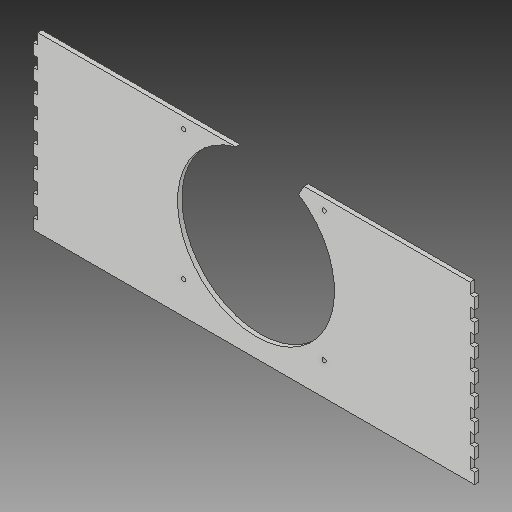
# Autodesk Inventor part: Stenka
Saved by Autodesk Inventor 2019 (Build 230136000, 136)
## iProperties
Created: 2022-06-29
Part Number: Stenka
Material: Типовые
Document SubType Name: Modeling
Designer: korsh
Density: 1 g/cm^3
Appearance: По умолчанию
Author: korsh
Autodesk Inventor part; units mm, degrees
ref_plane "YZ Plane" through (0, 0, 0) normal (1, 0, 0) x (0, 1, 0)
ref_plane "XZ Plane" through (0, 0, 0) normal (0, 1, 0) x (-1, 0, 0)
ref_plane "XY Plane" through (0, 0, 0) normal (0, 0, 1) x (1, 0, 0)
sketch "Эскиз1" plane through (0, 0, 0) normal (0, 0, 1) x (1, 0, 0)
  line L0 (-77, 69.9999) -> (-77, -70.0001) projected
  line L1 (-202, 69.9999) -> (198, 69.9999)
  line L2 (198, 69.9999) -> (198, -70.0001)
  line L3 (198, -70.0001) -> (-202, -70.0001)
  line L4 (-202, -70.0001) -> (-202, 69.9999)
  line L5 (73, -70.0001) -> (73, 69.9999) projected
  arc A0 (-18.8748, 69.9999) -> (-18.8744, -70.0001) centre (0, 0) ccw projected
  arc A1 (18.8744, -70.0001) -> (39.3067, 60.9199) centre (0, 0) ccw projected
  line L6 (44.4476, 69.9999) -> (36.592, 56.1251) projected
  line L7 (73, 69.9999) -> (44.4476, 69.9999) projected
  circle A2 centre (63, 59.9999) radius 2 projected
  circle A3 centre (-67, 59.9999) radius 2 projected
  circle A4 centre (-67, -60.0001) radius 2 projected
  circle A5 centre (63, -60.0001) radius 2 projected
  line L8 (44.4476, 69.9999) -> (73, 69.9999)
  point P0 (0, 0)
  dimension "d0" = 140
  dimension "d1" = 400
  dimension "d2" = 150
  dimension "d3" = 125
  constraints: 10 end point, 3 equal length, 1 horizontal, 1 perpendicular, 2 other
  measures "d0" distance of L3.end L1.start
  measures "d1" distance between parallel lines of L2 L4
  measures "d2" distance between parallel lines of L5 L0
  measures "d3" distance between parallel lines of L4 L0
extrude "Выдавливание1" add sketch "Эскиз1" along normal blind 4
sketch "Эскиз2" plane through (0, 0, 4) normal (0, 0, 1) x (1, 0, 0)
  line L0 (-202, -70.0001) -> (198, -70.0001) projected
  line L1 (198, -70.0001) -> (198, -90.0001)
  arc A0 (-18.8744, -70.0001) -> (18.8744, -70.0001) centre (0, 0) ccw projected
  line L2 (-202, -70.0001) -> (198, -70.0001) projected
  line L3 (-202, 69.9999) -> (-202, -70.0001) projected
  line L4 (-202, -70.0001) -> (-202, -90.0001)
  line L5 (-202, -90.0001) -> (198, -90.0001)
  point P0 (0, 0)
  dimension "d6" = 20
  constraints: 6 end point, 2 vertical, 1 perpendicular
  measures "d6" distance of L0.end L1.end
extrude "Выдавливание2" add sketch "Эскиз2" against normal blind 4
sketch "Эскиз3" plane through (0, 0, 4) normal (0, 0, 1) x (1, 0, 0)
  line L0 (198, 69.9999) -> (198, -90.0001) projected
  line L1 (-202, 69.9999) -> (-202, -90.0001) projected
  line L2 (198, -90.0001) -> (-202, -90.0001) projected
  line L3 (198, -90.0001) -> (202, -90.0001)
  line L4 (202, -90.0001) -> (202, -80.0001)
  line L5 (202, -80.0001) -> (198, -80.0001)
  line L6 (198, -80.0001) -> (198, -90.0001)
  line L7 (198, -70.0001) -> (202, -70.0001)
  line L8 (202, -70.0001) -> (202, -60.0001)
  line L9 (202, -60.0001) -> (198, -60.0001)
  line L10 (198, -60.0001) -> (198, -70.0001)
  line L11 (198, -50.0001) -> (202, -50.0001)
  line L12 (202, -50.0001) -> (202, -40.0001)
  line L13 (202, -40.0001) -> (198, -40.0001)
  line L14 (198, -40.0001) -> (198, -50.0001)
  line L15 (198, -30.0001) -> (202, -30.0001)
  line L16 (202, -30.0001) -> (202, -20.0001)
  line L17 (202, -20.0001) -> (198, -20.0001)
  line L18 (198, -20.0001) -> (198, -30.0001)
  line L19 (198, -10.0001) -> (202, -10.0001)
  line L20 (202, -10.0001) -> (202, -0.0001)
  line L21 (202, -0.0001) -> (198, -0.0001)
  line L22 (198, -0.0001) -> (198, -10.0001)
  line L23 (198, 9.9999) -> (202, 9.9999)
  line L24 (202, 9.9999) -> (202, 19.9999)
  line L25 (202, 19.9999) -> (198, 19.9999)
  line L26 (198, 19.9999) -> (198, 9.9999)
  line L27 (198, 29.9999) -> (202, 29.9999)
  line L28 (202, 29.9999) -> (202, 39.9999)
  line L29 (202, 39.9999) -> (198, 39.9999)
  line L30 (198, 39.9999) -> (198, 29.9999)
  line L31 (198, 49.9999) -> (202, 49.9999)
  line L32 (202, 49.9999) -> (202, 59.9999)
  line L33 (202, 59.9999) -> (198, 59.9999)
  line L34 (198, 59.9999) -> (198, 49.9999)
  line L35 (-202, -90.0001) -> (-206, -90.0001)
  line L36 (-206, -90.0001) -> (-206, -80.0001)
  line L37 (-206, -80.0001) -> (-202, -80.0001)
  line L38 (-202, -80.0001) -> (-202, -90.0001)
  line L39 (-206, -60.0001) -> (-202, -60.0001)
  line L40 (-202, -70.0001) -> (-206, -70.0001)
  line L41 (-206, -70.0001) -> (-206, -60.0001)
  line L42 (-202, -60.0001) -> (-202, -70.0001)
  line L43 (-206, -40.0001) -> (-202, -40.0001)
  line L44 (-202, -50.0001) -> (-206, -50.0001)
  line L45 (-206, -50.0001) -> (-206, -40.0001)
  line L46 (-202, -40.0001) -> (-202, -50.0001)
  line L47 (-206, -20.0001) -> (-202, -20.0001)
  line L48 (-202, -30.0001) -> (-206, -30.0001)
  line L49 (-206, -30.0001) -> (-206, -20.0001)
  line L50 (-202, -20.0001) -> (-202, -30.0001)
  line L51 (-206, -0.0001) -> (-202, -0.0001)
  line L52 (-202, -10.0001) -> (-206, -10.0001)
  line L53 (-206, -10.0001) -> (-206, -0.0001)
  line L54 (-202, -0.0001) -> (-202, -10.0001)
  line L55 (-206, 19.9999) -> (-202, 19.9999)
  line L56 (-202, 9.9999) -> (-206, 9.9999)
  line L57 (-206, 9.9999) -> (-206, 19.9999)
  line L58 (-202, 19.9999) -> (-202, 9.9999)
  line L59 (-206, 39.9999) -> (-202, 39.9999)
  line L60 (-202, 29.9999) -> (-206, 29.9999)
  line L61 (-206, 29.9999) -> (-206, 39.9999)
  line L62 (-202, 39.9999) -> (-202, 29.9999)
  line L63 (-206, 59.9999) -> (-202, 59.9999)
  line L64 (-202, 49.9999) -> (-206, 49.9999)
  line L65 (-206, 49.9999) -> (-206, 59.9999)
  line L66 (-202, 59.9999) -> (-202, 49.9999)
  point P0 (0, 0)
  dimension "d9" = 4
  dimension "d10" = 10
  dimension "d13" = 20
  dimension "d18" = 4
  dimension "d21" = 20
  constraints: 128 end point, 4 parallel, 2 horizontal, 2 perpendicular, 2 vertical, 112 other
  measures "d9" distance of L5.end L4.end
  measures "d10" distance of L4.end L3.end
  measures "d13" distance of L4.end L8.end
  measures "d18" distance of L36.end L37.end
  measures "d21" distance of L37.end L39.end
extrude "Выдавливание3" add sketch "Эскиз3" against normal blind 4
sketch "Эскиз4" plane through (0, 0, 4) normal (0, 0, 1) x (1, 0, 0)
  arc A0 (-18.8748, 69.9999) -> (-18.8744, -70.0001) centre (0, 0) ccw projected
  arc A1 (18.8744, -70.0001) -> (39.3067, 60.9199) centre (0, 0) ccw projected
  arc A2 (-18.8744, -70.0001) -> (18.8744, -70.0001) centre (0, 0) ccw projected
  line L0 (44.4476, 69.9999) -> (36.592, 56.1251) projected
  line L1 (198, 69.9999) -> (-202, 69.9999) projected
  point P0 (0, 0)
extrude "Выдавливание4" cut sketch "Эскиз4" against normal blind 4
equation "\"d3\" = -0.5 * d2 + 0.5 * d1"
